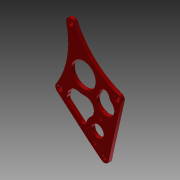
# Autodesk Inventor part: OutlineSketch1
Saved by Autodesk Inventor 2013 (Build 170138000, 138)
## iProperties
Created: 2013-06-03
Part Number: OutlineSketch1
Material: Aluminum 6061
Document SubType Name: Modeling
Designer: mvarma
Density: 1 g/cm^3
Author: mvarma
Autodesk Inventor part; units mm, degrees
ref_plane "YZ Plane" through (0, 0, 0) normal (1, 0, 0) x (0, 1, 0)
ref_plane "XZ Plane" through (0, 0, 0) normal (0, 1, 0) x (-1, 0, 0)
ref_plane "XY Plane" through (0, 0, 0) normal (0, 0, 1) x (1, 0, 0)
sketch "Sketch1" plane through (0, 0, 0) normal (0, 0, 1) x (1, 0, 0)
  line L0 (0, 0) -> (304.8, 0) construction
  line L1 (304.8, 0) -> (304.8, 50.8) construction
  line L2 (304.8, 50.8) -> (0, 50.8) construction
  line L3 (0, 50.8) -> (0, 0) construction
  circle A0 centre (152.4, 23.8125) radius 6.35 construction
  circle A1 centre (152.4, 23.8125) radius 34.29 construction
  circle A2 centre (152.4, 23.8125) radius 22.225 construction
  line L4 (152.4, 23.8125) -> (139.52, 61.741) construction
  circle A3 centre (139.52, 61.741) radius 9.525 construction
  circle A4 centre (139.52, 61.741) radius 17.78 construction
  circle A5 centre (91.5619, 85.09) radius 31.75 construction
  circle A6 centre (163.3424, 109.4657) radius 31.75 construction
  circle A7 centre (222.6465, 85.09) radius 31.75 construction
  line L5 (0, 50.8) -> (0, 53.34) construction
  line L6 (0, 53.34) -> (304.8, 53.34) construction
  line L7 (304.8, 53.34) -> (304.8, 50.8) construction
  circle A8 centre (139.52, 61.741) radius 21.59 construction
  circle A9 centre (152.4, 23.8125) radius 46.99 construction
  circle A10 centre (152.4, 23.8125) radius 50.8 construction
  arc A11 (86.3865, 79.4564) -> (92.4363, 92.6899) centre (91.5619, 85.09) ccw construction
  circle A12 centre (163.3424, 109.4657) radius 7.65 construction
  arc A13 (222.2546, 92.73) -> (226.29, 78.3634) centre (222.6465, 85.09) ccw construction
  circle A14 centre (163.3424, 109.4657) radius 9.1 construction
  circle A15 centre (139.52, 61.741) radius 22.9 construction
  line L8 (86.3865, 79.4564) -> (124.0276, 44.8769) construction
  line L9 (170.8782, 108.1486) -> (162.078, 57.7984) construction
  line L10 (92.4363, 92.6899) -> (91.5619, 85.09) construction
  line L11 (91.5619, 85.09) -> (86.3865, 79.4564) construction
  circle A16 centre (127.6738, 96.6252) radius 3.9688
  circle A17 centre (127.6738, 96.6252) radius 7.9375 construction
  line L12 (92.4363, 92.6899) -> (126.7664, 88.7398) construction
  line L13 (133.1953, 90.9229) -> (158.0208, 114.9615) construction
  line L14 (158.0208, 114.9615) -> (163.3424, 109.4657) construction
  line L15 (170.8782, 108.1486) -> (163.3424, 109.4657) construction
  line L16 (139.52, 61.741) -> (127.6738, 96.6252) construction
  line L17 (91.5619, 85.09) -> (163.3424, 109.4657) construction
  line L18 (152.4, 23.8125) -> (91.5619, 85.09) construction
  line L19 (152.4, 23.8125) -> (163.3424, 109.4657) construction
  circle A18 centre (127.6738, 96.6252) radius 9.2075 construction
  circle A19 centre (127.6738, 96.6252) radius 6.1595 construction
  arc A20 (92.4363, 92.6899) -> (86.3865, 79.4564) centre (91.5619, 85.09) ccw construction
  circle A21 centre (163.3424, 109.4657) radius 25.4 construction
  circle A22 centre (222.6465, 85.09) radius 25.4 construction
  line L20 (104.7627, 113.9656) -> (78.361, 56.2144) construction
  circle A23 centre (91.5619, 85.09) radius 25.4 construction
  line L21 (214.0607, 115.6571) -> (231.2324, 54.5229) construction
  line L22 (56.0019, 185.6657) -> (208.4019, 185.6657)
  line L23 (208.4019, 185.6657) -> (208.4019, -4.8343)
  line L24 (208.4019, -4.8343) -> (56.0019, -4.8343)
  line L25 (56.0019, -4.8343) -> (56.0019, 185.6657)
  circle A24 centre (139.52, 61.741) radius 11.1125
  arc A25 (226.1312, 75.4959) -> (221.6192, 95.3086) centre (223.8752, 85.4023) ccw construction
  line L26 (221.4349, 84.7168) -> (229.5152, 60.6363) construction
  line L27 (223.8752, 85.4023) -> (229.5152, 60.6363) construction
  line L28 (221.4349, 84.7168) -> (213.3547, 108.7973) construction
  line L29 (223.8752, 85.4023) -> (218.2352, 110.1682) construction
  arc A26 (212.5972, 111.0549) -> (214.1122, 106.5398) centre (213.3547, 108.7973) ccw construction
  arc A27 (218.764, 107.8464) -> (217.7065, 112.49) centre (218.2352, 110.1682) ccw construction
  arc A28 (218.764, 107.8464) -> (214.1122, 106.5398) centre (229.5152, 60.6363) ccw construction
  arc A29 (217.7065, 112.49) -> (212.5972, 111.0549) centre (229.5152, 60.6363) ccw construction
  line L30 (213.3547, 108.7973) -> (212.5972, 111.0549) construction
  line L31 (218.2352, 110.1682) -> (217.7065, 112.49) construction
  arc A30 (221.6192, 95.3086) -> (218.2029, 94.349) centre (229.5152, 60.6363) ccw construction
  arc A31 (226.1312, 75.4959) -> (224.667, 75.0846) centre (229.5152, 60.6363) ccw construction
  line L32 (104.4015, 107.0791) -> (92.7013, 84.5343) construction
  line L33 (81.0012, 61.9895) -> (90.3961, 85.5882) construction
  arc A32 (100.6718, 111.3992) -> (98.9102, 106.9744) centre (99.791, 109.1868) ccw construction
  arc A33 (103.3046, 104.9655) -> (105.4983, 109.1926) centre (104.4015, 107.0791) ccw construction
  arc A34 (103.3046, 104.9655) -> (98.9102, 106.9744) centre (81.0012, 61.9895) ccw construction
  line L34 (99.791, 109.1868) -> (100.6718, 111.3992) construction
  line L35 (104.4015, 107.0791) -> (105.4983, 109.1926) construction
  arc A35 (105.4983, 109.1926) -> (100.6718, 111.3992) centre (81.0012, 61.9895) ccw construction
  arc A36 (218.2029, 94.349) -> (224.667, 75.0846) centre (221.4349, 84.7168) ccw construction
  arc A37 (88.0213, 75.5164) -> (97.3814, 93.5522) centre (92.7013, 84.5343) ccw construction
  line L36 (90.3961, 85.5882) -> (99.791, 109.1868) construction
  line L37 (92.7013, 84.5343) -> (81.0012, 61.9895) construction
  arc A38 (88.0213, 75.5164) -> (86.6381, 76.1487) centre (81.0012, 61.9895) ccw construction
  arc A39 (97.3814, 93.5522) -> (94.1541, 95.0276) centre (81.0012, 61.9895) ccw construction
  arc A40 (94.1541, 95.0276) -> (86.6381, 76.1487) centre (90.3961, 85.5882) ccw construction
  line L38 (163.3424, 109.4657) -> (140.8985, 121.3583) construction
  line L39 (163.3424, 109.4657) -> (185.7862, 97.5731) construction
  circle A41 centre (139.52, 61.741) radius 26.71 construction
  line L40 (222.2546, 92.73) -> (138.1517, 88.4159) construction
  line L41 (226.29, 78.3634) -> (152.2412, 38.2549) construction
  line L42 (222.6465, 85.09) -> (222.2546, 92.73) construction
  line L43 (222.6465, 85.09) -> (226.29, 78.3634) construction
  line L44 (139.52, 61.741) -> (138.1517, 88.4159) construction
  line L45 (139.52, 61.741) -> (152.2412, 38.2549) construction
  arc A42 (226.29, 78.3634) -> (222.2546, 92.73) centre (222.6465, 85.09) ccw construction
  arc A43 (226.29, 78.3634) -> (225.5574, 78.0155) centre (222.6465, 85.09) ccw construction
  line L46 (139.52, 61.741) -> (222.6465, 85.09) construction
  circle A44 centre (139.52, 61.741) radius 15.875
  circle A45 centre (117.7793, 40.0955) radius 3.9688
  circle A46 centre (169.9459, 57.8106) radius 3.9688
  circle A47 centre (56.3388, 79.9803) radius 69.2823
  circle A48 centre (194.3931, 126.8617) radius 69.2823
  arc A49 (163.3226, 14.7011) -> (164.9427, 17.104) centre (152.4, 23.8125) ccw
  circle A50 centre (152.4, 23.8125) radius 11.176 construction
  circle A51 centre (152.4, 23.8125) radius 19.05 construction
  line L47 (115.1893, 37.0884) -> (143.1176, 13.0348)
  line L48 (152.4, 23.8125) -> (143.1176, 13.0348) construction
  line L49 (173.8315, 57.0025) -> (166.326, 20.9161) construction
  line L50 (152.4, 23.8125) -> (166.326, 20.9161) construction
  arc A52 (154.6674, 4.8437) -> (156.0456, 2.6757) centre (158.5256, 5.7742) ccw
  line L51 (152.4, 23.8125) -> (158.5256, 5.7742) construction
  arc A53 (156.9738, 10.3439) -> (163.3226, 14.7011) centre (152.4, 23.8125) ccw
  arc A54 (150.0325, 9.7869) -> (156.9738, 10.3439) centre (152.4, 23.8125) ccw
  arc A55 (157.2494, 9.5322) -> (154.6674, 4.8437) centre (158.5256, 5.7742) ccw
  arc A56 (162.061, 7.5775) -> (157.2494, 9.5322) centre (158.5256, 5.7742) ccw
  line L52 (143.5118, 12.7075) -> (156.0456, 2.6757)
  line L53 (162.3795, 4.8266) -> (166.2126, 20.4164) construction
  line L54 (143.5118, 12.7075) -> (152.4, 23.8125) construction
  line L55 (152.4, 23.8125) -> (166.2126, 20.4164) construction
  arc A57 (166.2126, 20.4164) -> (166.326, 20.9161) centre (152.4, 23.8125) ccw
  arc A58 (166.326, 20.9161) -> (166.6096, 24.4522) centre (152.4, 23.8125) ccw construction
  arc A59 (143.1176, 13.0348) -> (143.5118, 12.7075) centre (152.4, 23.8125) ccw
  arc A60 (143.5118, 12.7075) -> (150.0325, 9.7869) centre (152.4, 23.8125) ccw
  circle A61 centre (152.4, 23.8125) radius 5.5065
  line L56 (152.4, 23.8125) -> (166.2715, 20.6657)
  line L57 (166.6096, 24.4522) -> (164.9427, 17.104)
  arc A62 (164.9427, 17.104) -> (166.2126, 20.4164) centre (152.4, 23.8125) ccw construction
  line L58 (164.9427, 17.104) -> (162.4107, 4.9639)
  line L59 (158.5256, 5.7742) -> (162.4107, 4.9639) construction
  arc A63 (166.6096, 24.4522) -> (143.1176, 13.0348) centre (152.4, 23.8125) ccw
  line L60 (169.9459, 57.8106) -> (173.8204, 56.9509) construction
  line L61 (173.8204, 56.9509) -> (166.6096, 24.4522)
  line L62 (154.8725, 34.7116) -> (149.9275, 12.9134) construction
  circle A64 centre (154.8725, 34.7116) radius 2.1082
  circle A65 centre (149.9275, 12.9134) radius 2.1082
  arc A66 (162.4107, 4.9639) -> (162.061, 7.5775) centre (158.5256, 5.7742) ccw
  arc A67 (156.0456, 2.6757) -> (162.4107, 4.9639) centre (158.5256, 5.7742) ccw
  point P0 (215.7779, 109.5437)
  point P1 (102.1225, 108.1905)
  point P2 (145.0256, 46.8513)
  point P3 (171.2705, 61.5518)
  point P4 (114.4504, 42.2565)
  point P5 (131.2886, 98.2635)
  point P6 (123.8088, 95.7234)
  dimension "d127" = 31.75
  dimension "d150" = 38.1
  dimension "d1" = 50.8
  dimension "d3" = 23.8125
  dimension "d4" = 152.4
  dimension "d7" = 68.58
  dimension "d8" = 44.45
  dimension "d9" = 19.05
  dimension "d10" = 35.56
  dimension "d11" = 40.0558
  dimension "d12" = 63.5
  dimension "d13" = 63.5
  dimension "d14" = 63.5
  dimension "d15" = 2.54
  dimension "d16" = 304.8
  dimension "d17" = 43.18
  dimension "d18" = 93.98
  dimension "d19" = 101.6
  dimension "d21" = 15.3
  dimension "d22" = 15.3
  dimension "d24" = 18.2
  dimension "d29" = 45.8
  dimension "d30" = 143.991
  dimension "d31" = 7.9375
  dimension "d32" = 15.875
  dimension "d33" = 143.991
  dimension "d35" = 18.415
  dimension "d37" = 12.319
  dimension "d40" = 50.8
  dimension "d41" = 50.8
  dimension "d42" = 18.004
  dimension "d43" = 18.004
  dimension "d44" = 50.8
  dimension "d53" = 152.4
  dimension "d54" = 190.5
  dimension "d55" = 35.56
  dimension "d56" = 76.2
  dimension "d57" = 22.225
  dimension "d67" = 25.4
  dimension "d68" = 25.4
  dimension "d69" = 2.86
  dimension "d70" = 25.4
  dimension "d71" = 25.4
  dimension "d72" = 4.7625
  dimension "d75" = 2.86
  dimension "d80" = 4.7625
  dimension "d82" = 4.7625
  dimension "d83" = 50.8
  dimension "d84" = 50.8
  dimension "d85" = 10.16
  dimension "d97" = 48.4188
  dimension "d99" = 20.32
  dimension "d101" = 25.4
  dimension "d102" = 25.4
  dimension "d103" = 10.16
  dimension "d105" = 18.004
  dimension "d106" = 18.004
  dimension "d107" = 53.42
  dimension "d108" = 154.494
  dimension "d109" = 7.65
  dimension "d111" = 86.3435
  dimension "d112" = 12.753
  dimension "d113" = 12.753
  dimension "d135" = 7.9375
  dimension "d136" = 7.9375
  dimension "d149" = 22.352
  constraints: 130 end point, 112 point on circle, 66 centre point, 56 tangent, 41 coincident, 16 point on line, 14 perpendicular, 10 collinear, 8 parallel, 3 midpoint, 2 horizontal, 1 equal radius, 11 other
  measures "d1" distance of L1.end L0.end
  measures "d3" distance from line of L0 A0.centre
  measures "d4" distance from line of L3 A0.centre
  measures "d7" diameter of A1
  measures "d8" diameter of A2
  measures "d9" diameter of A3
  measures "d10" diameter of A4
  measures "d11" distance of L4.start L4.end
  measures "d12" diameter of A5
  measures "d13" diameter of A6
  measures "d14" diameter of A7
  measures "d15" distance of L2.end L5.end
  measures "d16" distance of L0.end L0.start
  measures "d17" diameter of A8
  measures "d18" diameter of A9
  measures "d19" diameter of A10
  measures "d21" diameter of A11
  measures "d22" diameter of A12
  measures "d24" diameter of A14
  measures "d29" diameter of A15
  measures "d30" angle of L11 L10
  measures "d31" diameter of A16
  measures "d32" diameter of A17
  measures "d33" angle of L15 L14
  measures "d35" diameter of A18
  measures "d37" diameter of A19
  measures "d40" diameter of A21
  measures "d41" diameter of A22
  measures "d42" angle of L10 L20
  measures "d43" angle of L11 L20
  measures "d44" diameter of A23
  measures "d53" distance of L23.end L24.end
  measures "d54" distance of L22.end L23.end
  measures "d55" distance from line of L25 A5.centre
  measures "d56" distance from line of L22 A6.centre
  measures "d57" diameter of A24
  measures "d67" distance of L26.start L26.end
  measures "d68" distance of L27.start L26.end
  measures "d69" angle of L21 L26
  measures "d70" distance of L26.start L28.end
  measures "d71" distance of L27.start L29.end
  measures "d72" diameter of A26
  measures "d75" angle of L20 L32
  measures "d80" diameter of A32
  measures "d82" diameter of A33
  measures "d83" distance of L33.start L36.end
  measures "d84" distance of L32.start L33.start
  measures "d85" radius of A25
  measures "d97" radius of A34
  measures "d99" diameter of A37
  measures "d101" distance of L33.start L33.end
  measures "d102" distance of L32.end L33.start
  measures "d103" radius of A40
  measures "d105" angle of L38 L14
  measures "d106" angle of L39 L15
  measures "d107" diameter of A41
  measures "d108" angle of L42 L43
  measures "d109" radius of A13
  measures "d111" distance of L44.start L42.start
  measures "d112" angle of L21 L42
  measures "d113" angle of L21 L43
  measures "d135" diameter of A45
  measures "d136" diameter of A46
  measures "d149" diameter of A50
extrude "Extrusion3" add sketch "Sketch1" along normal blind 3.175 contours A16 | A16 A48 A44 A47 | A48 A46 L61 A63 L47 A45 A47 A44 | A44 | A46 | A45 | L57 A49 A53 A54 A60 A59 A63 | A60 A54 A53 A49 L58 A66 A56 A55 A52 L52 | A52 A55 A56 A66 A67 | A64 | A65
hole "Hole3" at (81.0012, 61.9895, 0) at (229.5152, 60.6363, 0) at (185.7862, 97.5731, 0) at (215.7779, 109.5437, 0) at (117.7793, 40.0955, 0) at (169.9459, 57.8106, 0) at (127.6738, 96.6252, 0) direction (0, 0, 1) diameter 4.9784 end through all clearance for "Socket Head Cap Screw" size "#10" standard "Ansi Unified Screw Threads"
hole "Hole4" at (100.6718, 111.3992, 0) at (105.4983, 109.1926, 0) at (140.8985, 121.3583, 0) at (102.1225, 108.1905, 0) at (158.5256, 5.7742, 0) direction (0, 0, 1) diameter 3.6576 end through all clearance for "Flat Head Machine Screw (82)" size "#6" standard "Ansi Unified Screw Threads"
hole "Hole5" at (154.8725, 34.7116, 0) at (149.9275, 12.9134, 0) direction (0, 0, 1) diameter 2.9464 end through all clearance for "Socket Head Cap Screw" size "#4" standard "Ansi Unified Screw Threads"
fillet "Fillet2" radius 3.175 2 edges at (164.9427, 17.104, 1.5875) (166.6096, 24.4522, 1.5875)
sketch "Sketch3" plane through (0, 0, 3.175) normal (0, 0, 1) x (1, 0, 0)
  circle A0 centre (152.4, 23.8125) radius 5.5065 projected
  circle A1 centre (139.52, 61.741) radius 11.1125 projected
  circle A2 centre (117.7793, 40.0955) radius 2.4892 projected
  circle A3 centre (149.9275, 12.9134) radius 1.4732 projected
  circle A4 centre (154.8725, 34.7116) radius 1.4732 projected
  arc A5 (142.2903, 25.6144) -> (146.0422, 31.8766) centre (152.4, 23.8125) ccw
  circle A6 centre (154.8725, 34.7116) radius 6.2357
  arc A7 (125.0102, 39.5472) -> (124.4796, 37.322) centre (117.7793, 40.0955) ccw
  arc A8 (140.6237, 45.9044) -> (135.0642, 46.5042) centre (139.52, 61.741) ccw
  arc A9 (125.0102, 39.5472) -> (135.0642, 46.5042) centre (132.8558, 38.9523) ccw construction
  arc A10 (140.6237, 45.9044) -> (146.0422, 31.8766) centre (141.1708, 38.0554) ccw construction
  line L0 (117.7793, 40.0955) -> (125.3632, 33.6831)
  arc A11 (125.3632, 33.6831) -> (124.4796, 37.322) centre (127.4132, 36.1076) ccw construction
  arc A12 (137.1146, 23.747) -> (142.2903, 25.6144) centre (139.1646, 26.1715) ccw
  arc A13 (124.4796, 37.322) -> (125.3632, 33.6831) centre (127.4132, 36.1076) ccw
  arc A14 (135.0642, 46.5042) -> (125.0102, 39.5472) centre (132.8558, 38.9523) ccw
  arc A15 (124.4796, 37.322) -> (125.0102, 39.5472) centre (117.7793, 40.0955) ccw
  arc A16 (135.0642, 46.5042) -> (140.6237, 45.9044) centre (139.52, 61.741) ccw
  arc A17 (148.8146, 36.19) -> (140.6237, 45.9044) centre (141.1708, 38.0554) ccw
  arc A18 (146.0422, 31.8766) -> (148.8146, 36.19) centre (141.1708, 38.0554) ccw
  arc A19 (146.0422, 31.8766) -> (142.2903, 25.6144) centre (152.4, 23.8125) ccw
  arc A20 (142.2903, 25.6144) -> (137.1146, 23.747) centre (139.1646, 26.1715) ccw construction
  line L1 (137.1146, 23.747) -> (149.9275, 12.9134)
  line L2 (125.3632, 33.6831) -> (137.1146, 23.747)
  line L3 (166.6112, 24.4595) -> (173.8204, 56.9509) projected
  arc A21 (131.2886, 98.2635) -> (171.2705, 61.5518) centre (194.3931, 126.8617) ccw projected
  circle A22 centre (169.9459, 57.8106) radius 2.4892 projected
  arc A23 (152.5359, 52.6525) -> (156.6824, 40.6788) centre (158.9547, 48.1705) ccw
  arc A24 (156.6824, 40.6788) -> (152.5359, 52.6525) centre (158.9547, 48.1705) ccw construction
  circle A25 centre (169.9459, 57.8106) radius 7.2517
  arc A26 (154.581, 56.723) -> (162.8587, 56.2747) centre (158.6584, 55.3645) ccw construction
  arc A27 (162.8587, 56.2747) -> (154.581, 56.723) centre (158.6584, 55.3645) ccw
  arc A28 (165.1215, 52.3966) -> (157.3984, 40.4128) centre (160.3212, 47.0097) ccw construction
  line L4 (168.0799, 48.6677) -> (166.1231, 39.8486) construction
  arc A29 (166.1426, 51.2726) -> (165.1215, 52.3966) centre (160.3212, 47.0097) ccw
  arc A30 (157.3984, 40.4128) -> (166.1426, 51.2726) centre (160.3212, 47.0097) ccw
  point P0 (0, 0)
  dimension "d194" = 4.7625
  dimension "d195" = 4.7625
  dimension "d196" = 4.7625
  dimension "d197" = 4.7625
  dimension "d200" = 6.35
  dimension "d201" = 6.35
  dimension "d204" = 4.7625
  dimension "d205" = 4.7625
  dimension "d206" = 6.35
  dimension "d208" = 3.81
  constraints: 52 point on circle, 24 centre point, 21 tangent, 8 end point, 5 coincident, 1 equal radius, 1 parallel
  measures "d194" radial gap between concentric circles of A2 A7
  measures "d195" radial gap between concentric circles of A4 A6
  measures "d196" radial gap between concentric circles of A0 A5
  measures "d197" radial gap between concentric circles of A1 A8
  measures "d200" diameter of A11
  measures "d201" diameter of A12
  measures "d205" radial gap between concentric circles of A22 A25
  measures "d208" distance between parallel lines of L3 L4
extrude "Extrusion5" cut sketch "Sketch3" against normal through all contours A19 A12 L2 A13 A15 A14 A16 A17 A18 | A6 A23 A8 A27 A25 A29 A30
equation "\"d8\" = Gear35tPD"
equation "\"d9\" = Gear15tPD"
equation "\"d10\" = Gear28tPD"
equation "\"d11\" = 0.5 * Gear48tPD + 0.5 * Gear15tPD + MeshingClearance"
equation "\"d12\" = CimOD"
equation "\"d13\" = CimOD"
equation "\"d14\" = CimOD"
equation "\"d17\" = Gear28tPD + ClearanceDiameter"
equation "\"d18\" = WheelOD"
equation "\"d19\" = WheelClearance"
equation "\"Pulley48tPD\" = 45.8"
equation "\"Pulley19tPD\" = 18.2"
equation "\"Pulley16tPD\" = 15.3"
equation "\"Gear15tPD\" = 19.05"
equation "\"Gear35tPD\" = 44.45"
equation "\"Gear48tPD\" = 60.96"
equation "\"Gear28tPD\" = 35.56"
equation "\"BearingLargeOD\" = 28.575"
equation "\"BearingSmallOD\" = 22.225"
equation "\"MeshingClearance\" = 0.0508"
equation "\"CimOD\" = 63.5"
equation "\"WheelOD\" = 93.98"
equation "\"ClearanceDiameter\" = 7.62"
equation "\"WheelClearance\" = 101.6"
equation "\"TensioningBearingID\" = 6.35"
equation "\"TensioningBearingOD\" = 15.875"
equation "\"SpingClipClearance\" = 8.89"
equation "\"Pi\" = 79.79645"
equation "\"Pulley56tPD\" = 53.5"
equation "\"BearingXLargeOD\" = 34.925"
body "Solid3"
